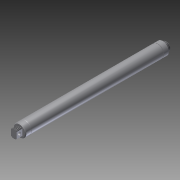
# Autodesk Inventor part: 6''  by 1'' dia piston
Saved by Autodesk Inventor 2012 (Build 160160000, 160)
## iProperties
Created: 2013-10-11
Part Number: 6''  by 1'' dia piston
Material: Default
Document SubType Name: Modeling
Designer: Bryce
Density: 1 g/cm^3
Author: Bryce
Autodesk Inventor part; units mm, degrees
ref_plane "YZ Plane" through (0, 0, 0) normal (1, 0, 0) x (0, 1, 0)
ref_plane "XZ Plane" through (0, 0, 0) normal (0, 1, 0) x (-1, 0, 0)
ref_plane "XY Plane" through (0, 0, 0) normal (0, 0, 1) x (1, 0, 0)
sketch "Sketch1" plane through (0, 0, 0) normal (0, 0, 1) x (1, 0, 0)
  circle A0 centre (0, 0) radius 12.7
  circle A1 centre (0, 0) radius 14.2875
  line L0 (-6.35, 7.0995) -> (6.35, 7.0995)
  line L1 (6.35, 7.0995) -> (6.35, -7.0995)
  line L2 (6.35, -7.0995) -> (-6.35, -7.0995)
  line L3 (-6.35, -7.0995) -> (-6.35, 7.0995)
  arc A2 (6.35, 7.0995) -> (-6.35, 7.0995) centre (0, 0) ccw
  arc A3 (-6.35, -7.0995) -> (6.35, -7.0995) centre (0, 0) ccw
  dimension "d2" = 25.4
  dimension "d3" = 28.575
  dimension "d4" = 12.7
  dimension "d5" = 6.35
  dimension "d6" = 14.199
  dimension "d7" = 7.0995
  dimension "d8" = 9.525
  constraints: 8 end point, 4 centre point, 4 point on circle, 3 coincident, 2 parallel, 1 concentric, 1 horizontal, 1 perpendicular
  measures "d2" diameter of A0
  measures "d3" diameter of A1
  measures "d4" distance of L0.start L0.end
  measures "d5" distance from line of L3 point (0, 0)
  measures "d6" distance of L0.end L1.end
  measures "d7" distance from line of L0 point (0, 0)
  measures "d8" radius of A2
extrude "Extrusion1" add sketch "Sketch1" against normal blind 304.8 contours A1
fillet "Fillet1" radius 0.7937 2 edges at (-14.2875, 0, 0) (-14.2875, 0, -304.8)
extrude "Extrusion2" add sketch "Sketch1" along normal blind 12.7 contours A0 | A1
extrude "Extrusion3" add sketch "Sketch1" along normal blind 25.4 contours A2 L0 | L0 L1 L2 L3 | L2 A3
chamfer "Chamfer1" distance 1.5875 angle 45 1 edges at (-14.2875, 0, 12.7)
thread "Thread1" size "3/4-10 UNC" class "2A" standard "ANSI Unified Screw Threads" full length
thread "Thread2" size "3/4-10 UNC" class "2A" standard "ANSI Unified Screw Threads" full length
sketch "Sketch2" plane through (0, 0, -304.8) normal (0, 0, -1) x (-1, 0, 0)
  circle A0 centre (0, 0) radius 14.2875 projected
  circle A1 centre (0, 0) radius 9.525
  circle A2 centre (0, 0) radius 3.175
  circle A3 centre (0, 0) radius 3.9688
  dimension "d24" = 19.05
  dimension "d25" = 7.9375
  dimension "d26" = 6.35
  constraints: 3 centre point, 3 coincident
  measures "d24" diameter of A1
  measures "d25" diameter of A3
  measures "d26" diameter of A2
extrude "Extrusion4" add sketch "Sketch2" along normal blind 12.7 contours A0
extrude "Extrusion5" add sketch "Sketch2" along normal blind 19.05 contours A3
fillet "Fillet2" radius 0.1905 2 edges at (3.9688, 0, -323.85) (3.175, 0, -323.85)
extrude "Extrusion6" add sketch "Sketch2" along normal blind 19.05 contours A1
chamfer "Chamfer2" distance 1.5875 angle 45 1 edges at (14.2875, 0, -317.5)
thread "Thread3" size "3/4-10 UNC" class "2A" standard "ANSI Unified Screw Threads" full length
sketch "Sketch3" plane through (6.35, -7.0995, 12.7) normal (1, 0, 0) x (0, 0, -1)
  line L0 (0, 14.199) -> (-12.7, 14.199) projected
  line L1 (-12.7, 14.199) -> (-12.7, 0) projected
  line L2 (0, 0) -> (-12.7, 0) projected
  circle A0 centre (-6.35, 7.0995) radius 3.175
  point P0 (12.7, 7.0995)
  dimension "d39" = 6.35
  dimension "d40" = 7.0995
  dimension "d41" = 14.199
  dimension "d42" = 6.35
  constraints: 1 centre point
  measures "d39" distance from line of L1 A0.centre
  measures "d40" distance from line of L0 A0.centre
  measures "d41" distance between parallel lines of L2 L0
  measures "d42" diameter of A0
extrude "Extrusion7" cut sketch "Sketch3" against normal blind 25.4
equation "\"d5\" = 0.5 * d4"
equation "\"d7\" = 0.5 * d6"
equation "\"d40\" = 0.5 * d41"
body "Solid1"
